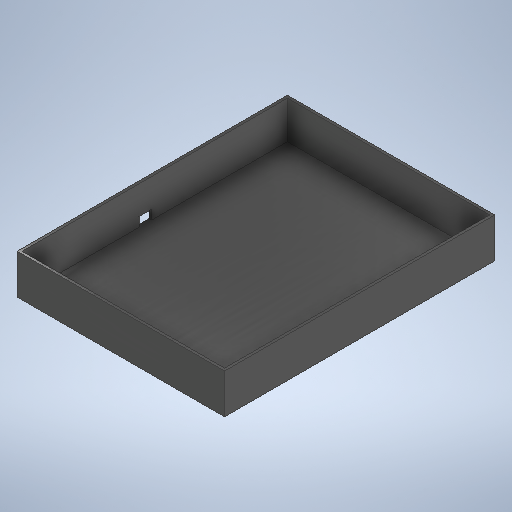
# Autodesk Inventor part: BaseFloor
Saved by Autodesk Inventor 2026.2 (Build 302298010, 298A)
## iProperties
Created: 2026-03-17
Part Number: BaseFloor
Material: Ogólny
Document SubType Name: Modeling
Designer: Patryk
Density: 1 g/cm^3
Appearance: Domyślna
Author: Patryk
Autodesk Inventor part; units mm, degrees
ref_plane "YZ Plane" through (0, 0, 0) normal (1, 0, 0) x (0, 1, 0)
ref_plane "XZ Plane" through (0, 0, 0) normal (0, 1, 0) x (-1, 0, 0)
ref_plane "XY Plane" through (0, 0, 0) normal (0, 0, 1) x (1, 0, 0)
sketch "Szkic1" plane through (0, 0, 0) normal (0, 1, 0) x (-1, 0, 0)
  line L0 (-165, -215) -> (165, -215)
  line L1 (165, -215) -> (165, 215)
  line L2 (165, 215) -> (-165, 215)
  line L3 (-165, 215) -> (-165, -215)
  line L4 (-165, -215) -> (165, 215) construction
  line L5 (165, -215) -> (-165, 215) construction
  point P0 (0, 0)
  dimension "d0" = 430
  dimension "d1" = 330
  constraints: 12 end point, 2 midpoint, 2 parallel, 1 horizontal, 1 perpendicular
  measures "d0" distance of L2.end L0.start
  measures "d1" distance of L1.end L2.end
extrude "Wyciągnięcie proste1" add sketch "Szkic1" along normal mid plane 3
sketch "Szkic2" plane through (0, 1.5, 0) normal (0, 1, 0) x (1, 0, 0)
  line L0 (161, -211) -> (-161, -211)
  line L1 (-161, -211) -> (-161, 211)
  line L2 (-161, 211) -> (161, 211)
  line L3 (161, 211) -> (161, -211)
  line L4 (161, -211) -> (-161, 211) construction
  line L5 (-161, -211) -> (161, 211) construction
  line L6 (-165, 215) -> (-165, -215) projected
  line L7 (-165, -215) -> (165, -215) projected
  line L8 (165, -215) -> (165, 215) projected
  line L9 (165, 215) -> (-165, 215) projected
  point P0 (0, 0)
  dimension "d4" = 322
  dimension "d5" = 422
  constraints: 12 end point, 2 midpoint, 2 parallel, 1 horizontal, 1 perpendicular
  measures "d4" distance between parallel lines of L3 L1
  measures "d5" distance between parallel lines of L0 L2
extrude "Wyciągnięcie proste2" add sketch "Szkic2" along normal blind 60
sketch "Szkic4" plane through (-165, -1.5, -215) normal (-1, 0, 0) x (0, 0, 1)
  line L0 (426, 3) -> (4, 3) projected
  line L1 (220, 3) -> (240, 3)
  line L2 (240, 3) -> (240, 18)
  line L3 (240, 18) -> (220, 18)
  line L4 (220, 18) -> (220, 3)
  line L5 (430, 0) -> (430, 63) projected
  point P0 (215, 1.5)
  dimension "d13" = 20
  dimension "d14" = 15
  dimension "d15" = 190
  constraints: 8 end point, 2 parallel, 1 horizontal, 1 perpendicular, 1 point on line
  measures "d13" distance of L2.end L3.end
  measures "d14" distance of L3.end L1.start
  measures "d15" distance between parallel lines of L5 L2
extrude "Wyciągnięcie proste4" cut sketch "Szkic4" against normal up to surface (4 mm away)
